Autodesk Fusion 360 part; units mm, degrees
note: some values were not read from the file. Set by a fixed rule: which sketch regions a step uses.
(part 6 of 8)
  spline S324 degree 3 poles (174.1756, -167.163) (173.9248, -167.1552) (173.6715, -167.2604) (173.4975, -167.451) knots 0 0 0 0 1 1 1 1
  spline S325 degree 3 poles (173.4975, -167.451) (173.3234, -167.6416) (173.2329, -167.9153) (173.2621, -168.1781) knots 0 0 0 0 1 1 1 1
  spline S326 degree 3 poles (173.2621, -168.1781) (173.2895, -168.4249) (173.4213, -168.6557) (173.6123, -168.8012) knots 0 0 0 0 1 1 1 1
  spline S327 degree 3 poles (173.6123, -168.8012) (173.8033, -168.9467) (174.0503, -169.0061) (174.283, -168.9676) knots 0 0 0 0 1 1 1 1
  spline S328 degree 3 poles (174.283, -168.9676) (174.4873, -168.9337) (174.6805, -168.8254) (174.8181, -168.6626) knots 0 0 0 0 1 1 1 1
  spline S329 degree 3 poles (174.8181, -168.6626) (174.9557, -168.4998) (175.036, -168.2834) (175.0353, -168.0653) knots 0 0 0 0 1 1 1 1
  spline S330 degree 3 poles (175.0353, -168.0653) (175.0345, -167.8296) (174.9387, -167.5967) (174.7791, -167.4316) knots 0 0 0 0 1 1 1 1
  spline S331 degree 3 poles (174.7791, -167.4316) (174.6196, -167.2666) (174.399, -167.1702) (174.1756, -167.163) knots 0 0 0 0 1 1 1 1
  spline S332 degree 3 poles (194.8527, -168.2399) (194.6019, -168.2321) (194.3486, -168.3373) (194.1746, -168.5279) knots 0 0 0 0 1 1 1 1
  spline S333 degree 3 poles (194.1746, -168.5279) (194.0006, -168.7185) (193.91, -168.9922) (193.9393, -169.255) knots 0 0 0 0 1 1 1 1
  spline S334 degree 3 poles (193.9393, -169.255) (193.9667, -169.5018) (194.0984, -169.7326) (194.2894, -169.8781) knots 0 0 0 0 1 1 1 1
  spline S335 degree 3 poles (194.2894, -169.8781) (194.4804, -170.0236) (194.7274, -170.083) (194.9602, -170.0445) knots 0 0 0 0 1 1 1 1
  spline S336 degree 3 poles (194.9602, -170.0445) (195.1645, -170.0106) (195.3576, -169.9023) (195.4953, -169.7395) knots 0 0 0 0 1 1 1 1
  spline S337 degree 3 poles (195.4953, -169.7395) (195.6328, -169.5767) (195.7131, -169.3603) (195.7124, -169.1422) knots 0 0 0 0 1 1 1 1
  spline S338 degree 3 poles (195.7124, -169.1422) (195.7117, -168.9065) (195.6158, -168.6736) (195.4563, -168.5085) knots 0 0 0 0 1 1 1 1
  spline S339 degree 3 poles (195.4563, -168.5085) (195.2967, -168.3435) (195.0761, -168.2471) (194.8527, -168.2399) knots 0 0 0 0 1 1 1 1
  spline S340 degree 3 poles (211.254, -162.4515) (211.0032, -162.4437) (210.75, -162.5489) (210.5759, -162.7395) knots 0 0 0 0 1 1 1 1
  spline S341 degree 3 poles (210.5759, -162.7395) (210.4019, -162.9302) (210.3114, -163.2038) (210.3406, -163.4666) knots 0 0 0 0 1 1 1 1
  spline S342 degree 3 poles (210.3406, -163.4666) (210.368, -163.7134) (210.4998, -163.9443) (210.6908, -164.0898) knots 0 0 0 0 1 1 1 1
  spline S343 degree 3 poles (210.6908, -164.0898) (210.8818, -164.2353) (211.1287, -164.2946) (211.3615, -164.2561) knots 0 0 0 0 1 1 1 1
  spline S344 degree 3 poles (211.3615, -164.2561) (211.5658, -164.2223) (211.759, -164.1139) (211.8966, -163.9511) knots 0 0 0 0 1 1 1 1
  spline S345 degree 3 poles (211.8966, -163.9511) (212.0342, -163.7884) (212.1144, -163.5719) (212.1137, -163.3538) knots 0 0 0 0 1 1 1 1
  spline S346 degree 3 poles (212.1137, -163.3538) (212.113, -163.1181) (212.0171, -162.8853) (211.8576, -162.7202) knots 0 0 0 0 1 1 1 1
  spline S347 degree 3 poles (211.8576, -162.7202) (211.698, -162.5551) (211.4774, -162.4587) (211.254, -162.4515) knots 0 0 0 0 1 1 1 1
  spline S348 degree 3 poles (210.4882, -175.711) (210.2374, -175.7031) (209.9841, -175.8083) (209.8101, -175.9989) knots 0 0 0 0 1 1 1 1
  spline S349 degree 3 poles (209.8101, -175.9989) (209.6361, -176.1896) (209.5455, -176.4632) (209.5748, -176.726) knots 0 0 0 0 1 1 1 1
  spline S350 degree 3 poles (209.5748, -176.726) (209.6022, -176.9728) (209.7339, -177.2037) (209.9249, -177.3492) knots 0 0 0 0 1 1 1 1
  spline S351 degree 3 poles (209.9249, -177.3492) (210.1159, -177.4947) (210.3629, -177.554) (210.5957, -177.5155) knots 0 0 0 0 1 1 1 1
  spline S352 degree 3 poles (210.5957, -177.5155) (210.8, -177.4817) (210.9931, -177.3733) (211.1307, -177.2106) knots 0 0 0 0 1 1 1 1
  spline S353 degree 3 poles (211.1307, -177.2106) (211.2683, -177.0478) (211.3486, -176.8313) (211.3479, -176.6132) knots 0 0 0 0 1 1 1 1
  spline S354 degree 3 poles (211.3479, -176.6132) (211.3471, -176.3775) (211.2513, -176.1447) (211.0917, -175.9796) knots 0 0 0 0 1 1 1 1
  spline S355 degree 3 poles (211.0917, -175.9796) (210.9322, -175.8145) (210.7116, -175.7181) (210.4882, -175.711) knots 0 0 0 0 1 1 1 1
  line L95 (197.7587, -166.6574) -> (197.7587, -165.3786)
  line L96 (197.7587, -165.3786) -> (207.3315, -165.6478)
  spline S356 degree 3 poles (207.3315, -165.6478) (208.1185, -165.9345) (208.8155, -166.489) (209.2929, -167.2084) knots 0 0 0 0 1 1 1 1
  spline S357 degree 3 poles (209.2929, -167.2084) (209.7704, -167.9277) (210.0258, -168.8082) (210.0119, -169.6862) knots 0 0 0 0 1 1 1 1
  spline S358 degree 3 poles (210.0119, -169.6862) (209.9996, -170.4556) (209.7819, -171.2202) (209.3902, -171.8694) knots 0 0 0 0 1 1 1 1
  spline S359 degree 3 poles (209.3902, -171.8694) (208.9984, -172.5186) (208.4339, -173.0505) (207.7782, -173.3881) knots 0 0 0 0 1 1 1 1
  line L97 (207.7782, -173.3881) -> (197.6949, -173.2534)
  line L98 (197.6949, -173.2534) -> (197.6311, -171.84)
  line L99 (197.6311, -171.84) -> (199.2904, -171.9073)
  line L100 (199.2904, -171.9073) -> (199.2904, -166.792)
  line L101 (199.2904, -166.792) -> (197.7587, -166.6574)
  line L102 (171.183, -170.5055) -> (171.183, -171.7666)
  line L103 (171.183, -171.7666) -> (161.8583, -171.5011)
  spline S360 degree 3 poles (161.8583, -171.5011) (161.0896, -171.2101) (160.4112, -170.6602) (159.9467, -169.9518) knots 0 0 0 0 1 1 1 1
  spline S361 degree 3 poles (159.9467, -169.9518) (159.4823, -169.2433) (159.2341, -168.3798) (159.2473, -167.5186) knots 0 0 0 0 1 1 1 1
  spline S362 degree 3 poles (159.2473, -167.5186) (159.259, -166.7632) (159.4705, -166.0123) (159.8517, -165.3727) knots 0 0 0 0 1 1 1 1
  spline S363 degree 3 poles (159.8517, -165.3727) (160.2329, -164.733) (160.7828, -164.2065) (161.4231, -163.8679) knots 0 0 0 0 1 1 1 1
  line L104 (161.4231, -163.8679) -> (171.2452, -164.0006)
  line L105 (171.2452, -164.0006) -> (171.3073, -165.3945)
  line L106 (171.3073, -165.3945) -> (169.691, -165.3281)
  line L107 (169.691, -165.3281) -> (169.691, -170.3727)
  line L108 (169.691, -170.3727) -> (171.183, -170.5055)
  spline S364 degree 3 poles (232.2093, -186.4811) (232.0787, -186.485) (231.9476, -186.4582) (231.8325, -186.4091) knots 0 0 0 0 1 1 1 1
  spline S365 degree 3 poles (231.8325, -186.4091) (231.7173, -186.3599) (231.6182, -186.2884) (231.5413, -186.2044) knots 0 0 0 0 1 1 1 1
  spline S366 degree 3 poles (231.5413, -186.2044) (231.3875, -186.0364) (231.3261, -185.8227) (231.3347, -185.6151) knots 0 0 0 0 1 1 1 1
  spline S367 degree 3 poles (231.3347, -185.6151) (231.3433, -185.4114) (231.4191, -185.2054) (231.5806, -185.0472) knots 0 0 0 0 1 1 1 1
  spline S368 degree 3 poles (231.5806, -185.0472) (231.6615, -184.9681) (231.7629, -184.9019) (231.8784, -184.8577) knots 0 0 0 0 1 1 1 1
  spline S369 degree 3 poles (231.8784, -184.8577) (231.994, -184.8134) (232.1236, -184.7917) (232.2515, -184.7986) knots 0 0 0 0 1 1 1 1
  spline S370 degree 3 poles (232.2515, -184.7986) (232.3753, -184.8054) (232.4962, -184.839) (232.6008, -184.892) knots 0 0 0 0 1 1 1 1
  spline S371 degree 3 poles (232.6008, -184.892) (232.7055, -184.945) (232.7941, -185.0172) (232.8622, -185.0997) knots 0 0 0 0 1 1 1 1
  spline S372 degree 3 poles (232.8622, -185.0997) (232.9984, -185.2647) (233.0502, -185.4674) (233.0418, -185.6646) knots 0 0 0 0 1 1 1 1
  spline S373 degree 3 poles (233.0418, -185.6646) (233.0332, -185.8575) (232.9676, -186.0524) (232.8236, -186.2078) knots 0 0 0 0 1 1 1 1
  spline S374 degree 3 poles (232.8236, -186.2078) (232.7516, -186.2855) (232.6607, -186.3525) (232.5554, -186.4006) knots 0 0 0 0 1 1 1 1
  spline S375 degree 3 poles (232.5554, -186.4006) (232.4502, -186.4488) (232.3307, -186.4778) (232.2093, -186.4811) knots 0 0 0 0 1 1 1 1
  line L109 (227.6589, -168.8588) -> (226.7503, -182.3862)
  spline S376 degree 3 poles (226.7503, -182.3862) (226.7201, -182.7001) (226.8342, -183.0214) (227.0661, -183.2766) knots 0 0 0 0 1 1 1 1
  spline S377 degree 3 poles (227.0661, -183.2766) (227.2917, -183.5246) (227.6269, -183.7085) (227.9987, -183.788) knots 0 0 0 0 1 1 1 1
  line L110 (227.9987, -183.788) -> (237.2483, -184.5544)
  spline S378 degree 3 poles (237.2483, -184.5544) (237.4241, -184.5476) (237.5976, -184.5046) (237.7473, -184.431) knots 0 0 0 0 1 1 1 1
  spline S379 degree 3 poles (237.7473, -184.431) (237.897, -184.3574) (238.0227, -184.2531) (238.1089, -184.1311) knots 0 0 0 0 1 1 1 1
  spline S380 degree 3 poles (238.1089, -184.1311) (238.261, -183.9159) (238.2873, -183.6607) (238.3138, -183.4147) knots 0 0 0 0 1 1 1 1
  spline S381 degree 3 poles (238.3138, -183.4147) (238.686, -179.9549) (239.0139, -176.4921) (239.2973, -173.0269) knots 0 0 0 0 1 1 1 1
  spline S382 degree 3 poles (239.2973, -173.0269) (239.6327, -168.9267) (239.9059, -164.8233) (240.1169, -160.7179) knots 0 0 0 0 1 1 1 1
  spline S383 degree 3 poles (240.1169, -160.7179) (240.1255, -160.5102) (240.0274, -160.3011) (239.8506, -160.148) knots 0 0 0 0 1 1 1 1
  spline S384 degree 3 poles (239.8506, -160.148) (239.668, -159.99) (239.4033, -159.8938) (239.1334, -159.8875) knots 0 0 0 0 1 1 1 1
  line L111 (239.1334, -159.8875) -> (229.1957, -159.4316)
  spline S385 degree 3 poles (229.1957, -159.4316) (228.874, -159.4703) (228.579, -159.6307) (228.4171, -159.855) knots 0 0 0 0 1 1 1 1
  spline S386 degree 3 poles (228.4171, -159.855) (228.3177, -159.9926) (228.2674, -160.1523) (228.2736, -160.3108) knots 0 0 0 0 1 1 1 1
  line L112 (228.2736, -160.3108) -> (228.1302, -163.0217)
  line L113 (228.1302, -163.0217) -> (227.157, -163.0339)
  spline S387 degree 3 poles (227.157, -163.0339) (227.062, -163.0349) (226.9664, -163.0378) (226.8736, -163.0542) knots 0 0 0 0 1 1 1 1
  spline S388 degree 3 poles (226.8736, -163.0542) (226.7809, -163.0707) (226.6916, -163.1005) (226.6139, -163.144) knots 0 0 0 0 1 1 1 1
  spline S389 degree 3 poles (226.6139, -163.144) (226.4429, -163.2396) (226.3333, -163.4012) (226.3271, -163.5673) knots 0 0 0 0 1 1 1 1
  line L114 (226.3271, -163.5673) -> (225.9787, -168.1425)
  spline S390 degree 3 poles (225.9787, -168.1425) (226.01, -168.2637) (226.0773, -168.3789) (226.1735, -168.4761) knots 0 0 0 0 1 1 1 1
  spline S391 degree 3 poles (226.1735, -168.4761) (226.2642, -168.5679) (226.3805, -168.6435) (226.5115, -168.6961) knots 0 0 0 0 1 1 1 1
  line L115 (226.5115, -168.6961) -> (227.6589, -168.8588)
  spline S392 degree 3 poles (224.9062, -160.356) (224.2581, -164.7818) (223.885, -169.233) (223.7889, -173.688) knots 0 0 0 0 1 1 1 1
  spline S393 degree 3 poles (223.7889, -173.688) (223.693, -178.1315) (223.8093, -182.576) (223.8307, -187.02) knots 0 0 0 0 1 1 1 1
  line L116 (223.8307, -187.02) -> (223.9723, -216.263)
  spline S394 degree 3 poles (223.9723, -216.263) (224.0231, -216.1601) (224.1235, -216.0732) (224.2482, -216.0243) knots 0 0 0 0 1 1 1 1
  spline S395 degree 3 poles (224.2482, -216.0243) (224.373, -215.9754) (224.5208, -215.965) (224.6544, -215.9957) knots 0 0 0 0 1 1 1 1
  spline S396 degree 3 poles (224.6544, -215.9957) (224.8058, -216.0304) (224.9345, -216.1157) (225.0202, -216.2207) knots 0 0 0 0 1 1 1 1
  spline S397 degree 3 poles (225.0202, -216.2207) (225.106, -216.3257) (225.151, -216.4494) (225.1677, -216.5739) knots 0 0 0 0 1 1 1 1
  spline S398 degree 3 poles (225.1677, -216.5739) (225.2012, -216.8228) (225.1259, -217.0718) (225.0962, -217.321) knots 0 0 0 0 1 1 1 1
  spline S399 degree 3 poles (225.0962, -217.321) (225.0221, -217.9422) (225.2425, -218.5829) (225.7041, -219.0877) knots 0 0 0 0 1 1 1 1
  spline S400 degree 3 poles (225.7041, -219.0877) (225.7417, -218.8946) (225.9077, -218.7202) (226.1313, -218.639) knots 0 0 0 0 1 1 1 1
  spline S401 degree 3 poles (226.1313, -218.639) (226.355, -218.5578) (226.6295, -218.5723) (226.8378, -218.6762) knots 0 0 0 0 1 1 1 1
  spline S402 degree 3 poles (226.8378, -218.6762) (226.9476, -218.7309) (227.0382, -218.8081) (227.1089, -218.8945) knots 0 0 0 0 1 1 1 1
  spline S403 degree 3 poles (227.1089, -218.8945) (227.1795, -218.9808) (227.2309, -219.0764) (227.2714, -219.1743) knots 0 0 0 0 1 1 1 1
  spline S404 degree 3 poles (227.2714, -219.1743) (227.3523, -219.3701) (227.3907, -219.5758) (227.4737, -219.771) knots 0 0 0 0 1 1 1 1
  spline S405 degree 3 poles (227.4737, -219.771) (227.6817, -220.261) (228.1819, -220.6668) (228.7939, -220.8424) knots 0 0 0 0 1 1 1 1
  spline S406 degree 3 poles (228.7939, -220.8424) (228.7215, -220.6271) (228.7391, -220.3931) (228.8436, -220.1862) knots 0 0 0 0 1 1 1 1
  spline S407 degree 3 poles (228.8436, -220.1862) (228.9481, -219.9793) (229.1387, -219.8005) (229.3783, -219.6846) knots 0 0 0 0 1 1 1 1
  spline S408 degree 3 poles (229.3783, -219.6846) (229.666, -219.5456) (230.0304, -219.5002) (230.3485, -219.588) knots 0 0 0 0 1 1 1 1
  spline S409 degree 3 poles (230.3485, -219.588) (230.5755, -219.6507) (230.7726, -219.7794) (230.894, -219.9442) knots 0 0 0 0 1 1 1 1
  spline S410 degree 3 poles (230.894, -219.9442) (231.0153, -220.109) (231.06, -220.3085) (231.0176, -220.4965) knots 0 0 0 0 1 1 1 1
  spline S411 degree 3 poles (231.0176, -220.4965) (231.399, -220.4565) (231.7539, -220.278) (231.9627, -220.0213) knots 0 0 0 0 1 1 1 1
  spline S412 degree 3 poles (231.9627, -220.0213) (232.1768, -219.758) (232.2327, -219.4363) (232.3304, -219.1326) knots 0 0 0 0 1 1 1 1
  spline S413 degree 3 poles (232.3304, -219.1326) (232.3792, -218.9807) (232.4403, -218.83) (232.537, -218.6934) knots 0 0 0 0 1 1 1 1
  spline S414 degree 3 poles (232.537, -218.6934) (232.6337, -218.5568) (232.7683, -218.4341) (232.94, -218.3571) knots 0 0 0 0 1 1 1 1
  spline S415 degree 3 poles (232.94, -218.3571) (233.1694, -218.2541) (233.4593, -218.2411) (233.7018, -218.3229) knots 0 0 0 0 1 1 1 1
  spline S416 degree 3 poles (233.7018, -218.3229) (233.9443, -218.4047) (234.1339, -218.5795) (234.2, -218.7821) knots 0 0 0 0 1 1 1 1
  spline S417 degree 3 poles (234.2, -218.7821) (234.4223, -218.5002) (234.5073, -218.1518) (234.4335, -217.8243) knots 0 0 0 0 1 1 1 1
  spline S418 degree 3 poles (234.4335, -217.8243) (234.3698, -217.5418) (234.196, -217.2842) (234.0477, -217.0225) knots 0 0 0 0 1 1 1 1
  spline S419 degree 3 poles (234.0477, -217.0225) (233.8994, -216.7608) (233.7726, -216.4781) (233.8125, -216.1929) knots 0 0 0 0 1 1 1 1
  spline S420 degree 3 poles (233.8125, -216.1929) (233.8482, -215.9371) (234.024, -215.6956) (234.2852, -215.5436) knots 0 0 0 0 1 1 1 1
  spline S421 degree 3 poles (234.2852, -215.5436) (234.5464, -215.3915) (234.8891, -215.3311) (235.2068, -215.3811) knots 0 0 0 0 1 1 1 1
  spline S422 degree 3 poles (235.2068, -215.3811) (235.2638, -215.0376) (235.1143, -214.676) (234.8118, -214.4264) knots 0 0 0 0 1 1 1 1
  spline S423 degree 3 poles (234.8118, -214.4264) (234.6592, -214.3006) (234.4734, -214.204) (234.2913, -214.1061) knots 0 0 0 0 1 1 1 1
  spline S424 degree 3 poles (234.2913, -214.1061) (234.1093, -214.0081) (233.9271, -213.906) (233.786, -213.7719) knots 0 0 0 0 1 1 1 1
  spline S425 degree 3 poles (233.786, -213.7719) (233.6493, -213.642) (233.555, -213.4842) (233.5148, -213.3179) knots 0 0 0 0 1 1 1 1
  spline S426 degree 3 poles (233.5148, -213.3179) (233.4745, -213.1516) (233.4885, -212.9772) (233.5549, -212.8163) knots 0 0 0 0 1 1 1 1
  spline S427 degree 3 poles (233.5549, -212.8163) (233.6212, -212.6554) (233.74, -212.5083) (233.8964, -212.3932) knots 0 0 0 0 1 1 1 1
  spline S428 degree 3 poles (233.8964, -212.3932) (234.0527, -212.2781) (234.2464, -212.1953) (234.4533, -212.155) knots 0 0 0 0 1 1 1 1
  spline S429 degree 3 poles (234.4533, -212.155) (234.3776, -211.9837) (234.2872, -211.8166) (234.183, -211.6551) knots 0 0 0 0 1 1 1 1
  spline S430 degree 3 poles (234.183, -211.6551) (233.5303, -210.6445) (232.3552, -209.8824) (231.7809, -208.8422) knots 0 0 0 0 1 1 1 1
  spline S431 degree 3 poles (231.7809, -208.8422) (231.2851, -207.944) (231.2866, -206.9141) (231.5335, -205.9531) knots 0 0 0 0 1 1 1 1
  spline S432 degree 3 poles (231.5335, -205.9531) (231.7803, -204.9922) (232.2581, -204.0804) (232.6953, -203.1633) knots 0 0 0 0 1 1 1 1
  spline S433 degree 3 poles (232.6953, -203.1633) (233.4614, -201.5562) (234.1092, -199.9155) (234.8011, -198.2873) knots 0 0 0 0 1 1 1 1
  spline S434 degree 3 poles (234.8011, -198.2873) (236.5126, -194.2596) (238.4993, -190.2944) (239.7468, -186.1605) knots 0 0 0 0 1 1 1 1
  spline S435 degree 3 poles (239.7468, -186.1605) (240.674, -183.0881) (241.1854, -179.9454) (241.5499, -176.7991) knots 0 0 0 0 1 1 1 1
  spline S436 degree 3 poles (241.5499, -176.7991) (242.1887, -171.2862) (242.3813, -165.7406) (242.1261, -160.2081) knots 0 0 0 0 1 1 1 1
  spline S437 degree 3 poles (242.1261, -160.2081) (241.9068, -158.8424) (241.1578, -157.5333) (240.0068, -156.5042) knots 0 0 0 0 1 1 1 1
  spline S438 degree 3 poles (240.0068, -156.5042) (238.8559, -155.4751) (237.3079, -154.7302) (235.6269, -154.3967) knots 0 0 0 0 1 1 1 1
  spline S439 degree 3 poles (235.6269, -154.3967) (233.2297, -153.9211) (230.5827, -154.3101) (228.5581, -155.4355) knots 0 0 0 0 1 1 1 1
  spline S440 degree 3 poles (228.5581, -155.4355) (226.5334, -156.5608) (225.1659, -158.4032) (224.9062, -160.356) knots 0 0 0 0 1 1 1 1
  spline S441 degree 3 poles (229.5936, -215.9494) (229.4411, -215.9533) (229.2882, -215.9209) (229.1557, -215.8607) knots 0 0 0 0 1 1 1 1
  spline S442 degree 3 poles (229.1557, -215.8607) (229.0232, -215.8006) (228.911, -215.7138) (228.8257, -215.6132) knots 0 0 0 0 1 1 1 1
  spline S443 degree 3 poles (228.8257, -215.6132) (228.6551, -215.4122) (228.5949, -215.1618) (228.6051, -214.9195) knots 0 0 0 0 1 1 1 1
  spline S444 degree 3 poles (228.6051, -214.9195) (228.6149, -214.6825) (228.6926, -214.4416) (228.8722, -214.2523) knots 0 0 0 0 1 1 1 1
  spline S445 degree 3 poles (228.8722, -214.2523) (228.962, -214.1576) (229.0766, -214.0771) (229.2091, -214.0227) knots 0 0 0 0 1 1 1 1
  spline S446 degree 3 poles (229.2091, -214.0227) (229.3417, -213.9683) (229.4924, -213.9406) (229.6412, -213.9484) knots 0 0 0 0 1 1 1 1
  spline S447 degree 3 poles (229.6412, -213.9484) (229.7862, -213.9562) (229.9273, -213.9972) (230.0477, -214.0618) knots 0 0 0 0 1 1 1 1
  spline S448 degree 3 poles (230.0477, -214.0618) (230.1682, -214.1263) (230.2683, -214.2137) (230.3437, -214.3124) knots 0 0 0 0 1 1 1 1
  spline S449 degree 3 poles (230.3437, -214.3124) (230.4944, -214.5098) (230.5443, -214.7476) (230.5344, -214.9783) knots 0 0 0 0 1 1 1 1
  spline S450 degree 3 poles (230.5344, -214.9783) (230.5246, -215.2032) (230.4579, -215.4317) (230.2981, -215.6175) knots 0 0 0 0 1 1 1 1
  spline S451 degree 3 poles (230.2981, -215.6175) (230.2182, -215.7104) (230.1156, -215.7916) (229.9949, -215.8505) knots 0 0 0 0 1 1 1 1
  spline S452 degree 3 poles (229.9949, -215.8505) (229.8742, -215.9093) (229.7351, -215.9453) (229.5936, -215.9494) knots 0 0 0 0 1 1 1 1
  spline S453 degree 3 poles (234.6434, -158.7579) (234.5128, -158.7618) (234.3817, -158.735) (234.2666, -158.6858) knots 0 0 0 0 1 1 1 1
  spline S454 degree 3 poles (234.2666, -158.6858) (234.1514, -158.6367) (234.0523, -158.5652) (233.9754, -158.4812) knots 0 0 0 0 1 1 1 1
  spline S455 degree 3 poles (233.9754, -158.4812) (233.8216, -158.3132) (233.7602, -158.0995) (233.7688, -157.8919) knots 0 0 0 0 1 1 1 1
  spline S456 degree 3 poles (233.7688, -157.8919) (233.7773, -157.6882) (233.8531, -157.4822) (234.0147, -157.324) knots 0 0 0 0 1 1 1 1
  spline S457 degree 3 poles (234.0147, -157.324) (234.0956, -157.2448) (234.197, -157.1787) (234.3125, -157.1345) knots 0 0 0 0 1 1 1 1
  spline S458 degree 3 poles (234.3125, -157.1345) (234.4281, -157.0902) (234.5576, -157.0685) (234.6855, -157.0754) knots 0 0 0 0 1 1 1 1
  spline S459 degree 3 poles (234.6855, -157.0754) (234.8094, -157.0822) (234.9303, -157.1158) (235.0349, -157.1688) knots 0 0 0 0 1 1 1 1
  spline S460 degree 3 poles (235.0349, -157.1688) (235.1395, -157.2218) (235.2282, -157.294) (235.2963, -157.3765) knots 0 0 0 0 1 1 1 1
  spline S461 degree 3 poles (235.2963, -157.3765) (235.4325, -157.5415) (235.4843, -157.7442) (235.4759, -157.9414) knots 0 0 0 0 1 1 1 1
  spline S462 degree 3 poles (235.4759, -157.9414) (235.4673, -158.1343) (235.4017, -158.3292) (235.2577, -158.4846) knots 0 0 0 0 1 1 1 1
  spline S463 degree 3 poles (235.2577, -158.4846) (235.1856, -158.5623) (235.0947, -158.6293) (234.9895, -158.6774) knots 0 0 0 0 1 1 1 1
  spline S464 degree 3 poles (234.9895, -158.6774) (234.8843, -158.7256) (234.7647, -158.7546) (234.6434, -158.7579) knots 0 0 0 0 1 1 1 1
  spline S465 degree 3 poles (227.5908, -200.8259) (227.6083, -200.9878) (227.7018, -201.1438) (227.8491, -201.2566) knots 0 0 0 0 1 1 1 1
  spline S466 degree 3 poles (227.8491, -201.2566) (227.9965, -201.3693) (228.1963, -201.4376) (228.4006, -201.4452) knots 0 0 0 0 1 1 1 1
  spline S467 degree 3 poles (228.4006, -201.4452) (228.5795, -201.452) (228.7607, -201.4123) (228.9102, -201.3339) knots 0 0 0 0 1 1 1 1
  spline S468 degree 3 poles (228.9102, -201.3339) (229.0597, -201.2555) (229.1767, -201.1387) (229.2393, -201.0054) knots 0 0 0 0 1 1 1 1
  line L117 (229.2393, -201.0054) -> (234.658, -188.8893)
  spline S469 degree 3 poles (234.658, -188.8893) (234.6959, -188.7185) (234.6569, -188.5375) (234.5495, -188.3865) knots 0 0 0 0 1 1 1 1
  spline S470 degree 3 poles (234.5495, -188.3865) (234.4371, -188.2285) (234.2507, -188.1047) (234.0351, -188.0448) knots 0 0 0 0 1 1 1 1
  line L118 (234.0351, -188.0448) -> (228.5617, -187.6122)
  spline S471 degree 3 poles (228.5617, -187.6122) (228.3722, -187.62) (228.1856, -187.6686) (228.0272, -187.7515) knots 0 0 0 0 1 1 1 1
  spline S472 degree 3 poles (228.0272, -187.7515) (227.7632, -187.8896) (227.5834, -188.1247) (227.5506, -188.3745) knots 0 0 0 0 1 1 1 1
  line L119 (227.5506, -188.3745) -> (227.5908, -200.8259)
  spline S473 degree 2 poles (42.2868, -37.3357) (44.6679, -37.1866) (46.1459, -37.3643) knots 0 0 0 1 1 1
  spline S474 degree 3 poles (46.1459, -37.3643) (46.1336, -38.9702) (46.0073, -41.0582) (46.5437, -41.5833) knots 0 0 0 0 1 1 1 1
  spline S475 degree 3 poles (46.5437, -41.5833) (47.2829, -42.5159) (49.4597, -43.7479) (51.759, -43.5945) knots 0 0 0 0 1 1 1 1
  spline S476 degree 3 poles (51.759, -43.5945) (54.1673, -43.434) (55.5304, -41.4405) (56.3952, -39.8243) knots 0 0 0 0 1 1 1 1
  spline S477 degree 3 poles (56.3952, -39.8243) (56.9698, -38.7504) (57.0179, -37.2523) (56.5268, -36.3258) knots 0 0 0 0 1 1 1 1
  spline S478 degree 3 poles (56.5268, -36.3258) (55.3043, -34.0192) (51.084, -30.618) (49.2463, -30.5751) knots 0 0 0 0 1 1 1 1
  spline S479 degree 3 poles (49.2463, -30.5751) (48.0943, -30.5466) (47.0495, -32.7405) (46.6501, -32.6627) knots 0 0 0 0 1 1 1 1
  spline S480 degree 3 poles (46.6501, -32.6627) (46.1834, -32.5719) (45.859, -32.1982) (45.6061, -31.8739) knots 0 0 0 0 1 1 1 1
  spline S481 degree 3 poles (45.6061, -31.8739) (45.2986, -31.4794) (47.8159, -29.3975) (47.8997, -28.7658) knots 0 0 0 0 1 1 1 1
  spline S482 degree 3 poles (47.8997, -28.7658) (47.9763, -28.1886) (47.7958, -27.8125) (47.6265, -27.6679) knots 0 0 0 0 1 1 1 1
  spline S483 degree 3 poles (47.6265, -27.6679) (47.2928, -27.3826) (46.6003, -27.122) (46.2027, -27.1804) knots 0 0 0 0 1 1 1 1
  spline S484 degree 3 poles (46.2027, -27.1804) (46.082, -27.1966) (45.9466, -27.2692) (45.9156, -27.3633) knots 0 0 0 0 1 1 1 1
  spline S485 degree 2 poles (45.9156, -27.3633) (45.8555, -27.5459) (45.85, -28.5927) knots 0 0 0 1 1 1
  line L120 (45.85, -28.5927) -> (42.3251, -28.6791)
  spline S486 degree 2 poles (42.3251, -28.6791) (42.2543, -27.7829) (42.0973, -27.3008) knots 0 0 0 1 1 1
  spline S487 degree 3 poles (42.0973, -27.3008) (42.0592, -27.1835) (41.8946, -27.0914) (41.7444, -27.0686) knots 0 0 0 0 1 1 1 1
  spline S488 degree 3 poles (41.7444, -27.0686) (41.511, -27.0319) (40.8, -27.289) (40.5387, -27.5865) knots 0 0 0 0 1 1 1 1
  spline S489 degree 3 poles (40.5387, -27.5865) (40.291, -27.8684) (40.33, -28.2666) (40.3538, -28.6072) knots 0 0 0 0 1 1 1 1
  spline S490 degree 3 poles (40.3538, -28.6072) (40.399, -29.2553) (43.1675, -31.4738) (42.9159, -31.8178) knots 0 0 0 0 1 1 1 1
  spline S491 degree 2 poles (42.9159, -31.8178) (42.6515, -32.1792) (41.8279, -32.7271) knots 0 0 0 1 1 1
  spline S492 degree 2 poles (41.8279, -32.7271) (40.3643, -30.4802) (39.2074, -30.5073) knots 0 0 0 1 1 1
  spline S493 degree 3 poles (39.2074, -30.5073) (38.2501, -30.5317) (33.4532, -34.048) (32.5474, -35.699) knots 0 0 0 0 1 1 1 1
  spline S494 degree 3 poles (32.5474, -35.699) (31.3187, -37.9383) (32.5495, -39.9259) (33.0916, -40.7431) knots 0 0 0 0 1 1 1 1
  spline S495 degree 3 poles (33.0916, -40.7431) (33.3686, -41.1607) (35.2173, -43.5307) (37.8353, -43.5361) knots 0 0 0 0 1 1 1 1
  spline S496 degree 3 poles (37.8353, -43.5361) (40.1284, -43.2704) (41.4838, -42.2707) (42.1123, -41.7993) knots 0 0 0 0 1 1 1 1
  spline S497 degree 3 poles (42.1123, -41.7993) (42.6989, -41.3593) (42.2945, -39.3731) (42.2867, -37.3353) knots 0 0 0 0 1 1 1 1
  line L121 (42.2867, -37.3353) -> (42.2868, -37.3357)
  spline S498 degree 3 poles (38.3817, -32.5359) (38.128, -32.5328) (37.8418, -32.7612) (37.8435, -32.9618) knots 0 0 0 0 1 1 1 1
  spline S499 degree 3 poles (37.8435, -32.9618) (37.8452, -33.1611) (38.1328, -33.3804) (38.3844, -33.3784) knots 0 0 0 0 1 1 1 1
  spline S500 degree 3 poles (38.3844, -33.3784) (38.6272, -33.3765) (38.8935, -33.1604) (38.8963, -32.9682) knots 0 0 0 0 1 1 1 1
  spline S501 degree 3 poles (38.8963, -32.9682) (38.8992, -32.7702) (38.6318, -32.5388) (38.3817, -32.5359) knots 0 0 0 0 1 1 1 1
  spline S502 degree 3 poles (40.6148, -34.9125) (40.3611, -34.9095) (40.0749, -35.1378) (40.0766, -35.3385) knots 0 0 0 0 1 1 1 1
  spline S503 degree 3 poles (40.0766, -35.3385) (40.0783, -35.5377) (40.3659, -35.757) (40.6175, -35.755) knots 0 0 0 0 1 1 1 1
  spline S504 degree 3 poles (40.6175, -35.755) (40.8602, -35.7531) (41.1266, -35.5371) (41.1294, -35.3449) knots 0 0 0 0 1 1 1 1
  spline S505 degree 3 poles (41.1294, -35.3449) (41.1323, -35.1469) (40.8649, -34.9154) (40.6148, -34.9125) knots 0 0 0 0 1 1 1 1
  spline S506 degree 3 poles (38.3, -34.8692) (38.0463, -34.8662) (37.7601, -35.0946) (37.7618, -35.2953) knots 0 0 0 0 1 1 1 1
  spline S507 degree 3 poles (37.7618, -35.2953) (37.7635, -35.4945) (38.0512, -35.7138) (38.3027, -35.7118) knots 0 0 0 0 1 1 1 1
  spline S508 degree 3 poles (38.3027, -35.7118) (38.5455, -35.7099) (38.8118, -35.4938) (38.8147, -35.3017) knots 0 0 0 0 1 1 1 1
  spline S509 degree 3 poles (38.8147, -35.3017) (38.8176, -35.1036) (38.5501, -34.8722) (38.3, -34.8692) knots 0 0 0 0 1 1 1 1
  spline S510 degree 3 poles (35.8218, -34.6316) (35.5681, -34.6286) (35.2819, -34.8569) (35.2837, -35.0576) knots 0 0 0 0 1 1 1 1
  spline S511 degree 3 poles (35.2837, -35.0576) (35.2854, -35.2569) (35.573, -35.4762) (35.8245, -35.4742) knots 0 0 0 0 1 1 1 1
  spline S512 degree 3 poles (35.8245, -35.4742) (36.0673, -35.4723) (36.3336, -35.2562) (36.3365, -35.064) knots 0 0 0 0 1 1 1 1
  spline S513 degree 3 poles (36.3365, -35.064) (36.3394, -34.866) (36.072, -34.6346) (35.8218, -34.6316) knots 0 0 0 0 1 1 1 1
  spline S514 degree 3 poles (36.2848, -37.6565) (36.0311, -37.6534) (35.7449, -37.8818) (35.7466, -38.0825) knots 0 0 0 0 1 1 1 1
  spline S515 degree 3 poles (35.7466, -38.0825) (35.7483, -38.2817) (36.0359, -38.501) (36.2875, -38.499) knots 0 0 0 0 1 1 1 1
  spline S516 degree 3 poles (36.2875, -38.499) (36.5303, -38.4972) (36.7966, -38.2811) (36.7995, -38.089) knots 0 0 0 0 1 1 1 1
  spline S517 degree 3 poles (36.7995, -38.089) (36.8023, -37.8909) (36.5349, -37.6595) (36.2848, -37.6565) knots 0 0 0 0 1 1 1 1
  spline S518 degree 3 poles (38.5723, -37.6996) (38.3186, -37.6966) (38.0324, -37.9249) (38.0342, -38.1256) knots 0 0 0 0 1 1 1 1
  spline S519 degree 3 poles (38.0342, -38.1256) (38.0358, -38.3249) (38.3235, -38.5442) (38.575, -38.5422) knots 0 0 0 0 1 1 1 1
  spline S520 degree 3 poles (38.575, -38.5422) (38.8178, -38.5403) (39.0841, -38.3242) (39.087, -38.132) knots 0 0 0 0 1 1 1 1
  spline S521 degree 3 poles (39.087, -38.132) (39.0899, -37.934) (38.8225, -37.7026) (38.5723, -37.6996) knots 0 0 0 0 1 1 1 1
  spline S522 degree 3 poles (40.996, -37.5052) (40.7423, -37.5022) (40.4561, -37.7305) (40.4579, -37.9312) knots 0 0 0 0 1 1 1 1
  spline S523 degree 3 poles (40.4579, -37.9312) (40.4596, -38.1305) (40.7472, -38.3498) (40.9987, -38.3478) knots 0 0 0 0 1 1 1 1
  spline S524 degree 3 poles (40.9987, -38.3478) (41.2415, -38.3459) (41.5078, -38.1298) (41.5107, -37.9376) knots 0 0 0 0 1 1 1 1
  spline S525 degree 3 poles (41.5107, -37.9376) (41.5136, -37.7396) (41.2462, -37.5082) (40.996, -37.5052) knots 0 0 0 0 1 1 1 1
  spline S526 degree 3 poles (34.0245, -37.2027) (33.7708, -37.1996) (33.4846, -37.428) (33.4863, -37.6287) knots 0 0 0 0 1 1 1 1
  spline S527 degree 3 poles (33.4863, -37.6287) (33.488, -37.8279) (33.7756, -38.0472) (34.0272, -38.0452) knots 0 0 0 0 1 1 1 1
  spline S528 degree 3 poles (34.0272, -38.0452) (34.27, -38.0433) (34.5363, -37.8273) (34.5391, -37.6351) knots 0 0 0 0 1 1 1 1
  spline S529 degree 3 poles (34.5391, -37.6351) (34.542, -37.4371) (34.2746, -37.2057) (34.0245, -37.2027) knots 0 0 0 0 1 1 1 1
  spline S530 degree 3 poles (35.7946, -40.3572) (35.5409, -40.3542) (35.2547, -40.5825) (35.2564, -40.7832) knots 0 0 0 0 1 1 1 1
  spline S531 degree 3 poles (35.2564, -40.7832) (35.2581, -40.9824) (35.5457, -41.2017) (35.7973, -41.1997) knots 0 0 0 0 1 1 1 1
  spline S532 degree 3 poles (35.7973, -41.1997) (36.0401, -41.1978) (36.3064, -40.9817) (36.3092, -40.7896) knots 0 0 0 0 1 1 1 1
  spline S533 degree 3 poles (36.3092, -40.7896) (36.3122, -40.5915) (36.0447, -40.3601) (35.7946, -40.3572) knots 0 0 0 0 1 1 1 1
  spline S534 degree 3 poles (37.9187, -40.3356) (37.665, -40.3325) (37.3788, -40.5609) (37.3806, -40.7616) knots 0 0 0 0 1 1 1 1
  spline S535 degree 3 poles (37.3806, -40.7616) (37.3823, -40.9609) (37.6699, -41.1801) (37.9214, -41.1782) knots 0 0 0 0 1 1 1 1
  spline S536 degree 3 poles (37.9214, -41.1782) (38.1642, -41.1762) (38.4305, -40.9602) (38.4334, -40.768) knots 0 0 0 0 1 1 1 1
  spline S537 degree 3 poles (38.4334, -40.768) (38.4363, -40.57) (38.1689, -40.3386) (37.9187, -40.3356) knots 0 0 0 0 1 1 1 1
  spline S538 degree 3 poles (40.3424, -39.9467) (40.0888, -39.9436) (39.8025, -40.172) (39.8043, -40.3726) knots 0 0 0 0 1 1 1 1
  spline S539 degree 3 poles (39.8043, -40.3726) (39.806, -40.5719) (40.0936, -40.7912) (40.3452, -40.7892) knots 0 0 0 0 1 1 1 1
  spline S540 degree 3 poles (40.3452, -40.7892) (40.5879, -40.7873) (40.8542, -40.5712) (40.8571, -40.379) knots 0 0 0 0 1 1 1 1
  spline S541 degree 3 poles (40.8571, -40.379) (40.86, -40.181) (40.5926, -39.9496) (40.3424, -39.9467) knots 0 0 0 0 1 1 1 1
  spline S542 degree 3 poles (49.8194, -32.5575) (49.5657, -32.5544) (49.2795, -32.7828) (49.2813, -32.9835) knots 0 0 0 0 1 1 1 1
  spline S543 degree 3 poles (49.2813, -32.9835) (49.2829, -33.1827) (49.5706, -33.402) (49.8221, -33.4) knots 0 0 0 0 1 1 1 1
  spline S544 degree 3 poles (49.8221, -33.4) (50.0649, -33.3981) (50.3312, -33.1821) (50.3341, -32.9899) knots 0 0 0 0 1 1 1 1
  spline S545 degree 3 poles (50.3341, -32.9899) (50.337, -32.7919) (50.0696, -32.5604) (49.8194, -32.5575) knots 0 0 0 0 1 1 1 1
  spline S546 degree 3 poles (47.4774, -34.8477) (47.2237, -34.8446) (46.9375, -35.073) (46.9392, -35.2736) knots 0 0 0 0 1 1 1 1
  spline S547 degree 3 poles (46.9392, -35.2736) (46.9409, -35.4729) (47.2286, -35.6922) (47.4801, -35.6902) knots 0 0 0 0 1 1 1 1
  spline S548 degree 3 poles (47.4801, -35.6902) (47.7229, -35.6883) (47.9892, -35.4722) (47.9921, -35.28) knots 0 0 0 0 1 1 1 1
  spline S549 degree 3 poles (47.9921, -35.28) (47.995, -35.082) (47.7275, -34.8506) (47.4774, -34.8477) knots 0 0 0 0 1 1 1 1
  spline S550 degree 3 poles (49.9011, -34.8692) (49.6474, -34.8662) (49.3612, -35.0946) (49.3629, -35.2953) knots 0 0 0 0 1 1 1 1
  spline S551 degree 3 poles (49.3629, -35.2953) (49.3646, -35.4945) (49.6522, -35.7138) (49.9038, -35.7118) knots 0 0 0 0 1 1 1 1
  spline S552 degree 3 poles (49.9038, -35.7118) (50.1466, -35.7099) (50.4129, -35.4938) (50.4158, -35.3017) knots 0 0 0 0 1 1 1 1
  spline S553 degree 3 poles (50.4158, -35.3017) (50.4187, -35.1036) (50.1512, -34.8722) (49.9011, -34.8692) knots 0 0 0 0 1 1 1 1
  spline S554 degree 3 poles (52.0252, -34.6748) (51.7716, -34.6718) (51.4853, -34.9001) (51.4871, -35.1008) knots 0 0 0 0 1 1 1 1
  spline S555 degree 3 poles (51.4871, -35.1008) (51.4888, -35.3) (51.7764, -35.5193) (52.028, -35.5173) knots 0 0 0 0 1 1 1 1
  spline S556 degree 3 poles (52.028, -35.5173) (52.2707, -35.5154) (52.537, -35.2994) (52.5399, -35.1072) knots 0 0 0 0 1 1 1 1
  spline S557 degree 3 poles (52.5399, -35.1072) (52.5428, -34.9092) (52.2754, -34.6778) (52.0252, -34.6748) knots 0 0 0 0 1 1 1 1
  spline S558 degree 3 poles (47.2868, -37.462) (47.0331, -37.4589) (46.7469, -37.6873) (46.7486, -37.8879) knots 0 0 0 0 1 1 1 1
  spline S559 degree 3 poles (46.7486, -37.8879) (46.7503, -38.0872) (47.0379, -38.3065) (47.2895, -38.3045) knots 0 0 0 0 1 1 1 1
  spline S560 degree 3 poles (47.2895, -38.3045) (47.5322, -38.3026) (47.7986, -38.0865) (47.8014, -37.8943) knots 0 0 0 0 1 1 1 1
  spline S561 degree 3 poles (47.8014, -37.8943) (47.8043, -37.6963) (47.5369, -37.4649) (47.2868, -37.462) knots 0 0 0 0 1 1 1 1
  spline S562 degree 3 poles (47.8586, -39.7738) (47.605, -39.7708) (47.3187, -39.9992) (47.3205, -40.1998) knots 0 0 0 0 1 1 1 1
  spline S563 degree 3 poles (47.3205, -40.1998) (47.3222, -40.3991) (47.6098, -40.6183) (47.8614, -40.6164) knots 0 0 0 0 1 1 1 1
  spline S564 degree 3 poles (47.8614, -40.6164) (48.1041, -40.6144) (48.3704, -40.3984) (48.3733, -40.2062) knots 0 0 0 0 1 1 1 1
  spline S565 degree 3 poles (48.3733, -40.2062) (48.3762, -40.0082) (48.1088, -39.7768) (47.8586, -39.7738) knots 0 0 0 0 1 1 1 1
  spline S566 degree 3 poles (49.7105, -37.678) (49.4568, -37.675) (49.1706, -37.9034) (49.1723, -38.1041) knots 0 0 0 0 1 1 1 1
  spline S567 degree 3 poles (49.1723, -38.1041) (49.174, -38.3033) (49.4616, -38.5226) (49.7132, -38.5206) knots 0 0 0 0 1 1 1 1
  spline S568 degree 3 poles (49.7132, -38.5206) (49.956, -38.5187) (50.2223, -38.3026) (50.2252, -38.1105) knots 0 0 0 0 1 1 1 1
  spline S569 degree 3 poles (50.2252, -38.1105) (50.228, -37.9124) (49.9606, -37.681) (49.7105, -37.678) knots 0 0 0 0 1 1 1 1
  spline S570 degree 3 poles (49.7105, -37.678) (49.4568, -37.675) (49.1706, -37.9034) (49.1723, -38.1041) knots 0 0 0 0 1 1 1 1
  spline S571 degree 3 poles (49.1723, -38.1041) (49.174, -38.3033) (49.4616, -38.5226) (49.7132, -38.5206) knots 0 0 0 0 1 1 1 1
  spline S572 degree 3 poles (49.7132, -38.5206) (49.956, -38.5187) (50.2223, -38.3026) (50.2252, -38.1105) knots 0 0 0 0 1 1 1 1
  spline S573 degree 3 poles (50.2252, -38.1105) (50.228, -37.9124) (49.9606, -37.681) (49.7105, -37.678) knots 0 0 0 0 1 1 1 1
  spline S574 degree 3 poles (50.0373, -40.4652) (49.7836, -40.4622) (49.4974, -40.6905) (49.4991, -40.8912) knots 0 0 0 0 1 1 1 1
  spline S575 degree 3 poles (49.4991, -40.8912) (49.5008, -41.0905) (49.7884, -41.3098) (50.04, -41.3078) knots 0 0 0 0 1 1 1 1
  spline S576 degree 3 poles (50.04, -41.3078) (50.2828, -41.3059) (50.5491, -41.0898) (50.5519, -40.8976) knots 0 0 0 0 1 1 1 1
  spline S577 degree 3 poles (50.5519, -40.8976) (50.5548, -40.6996) (50.2874, -40.4681) (50.0373, -40.4652) knots 0 0 0 0 1 1 1 1
  spline S578 degree 3 poles (52.5699, -40.4436) (52.3162, -40.4406) (52.03, -40.669) (52.0317, -40.8696) knots 0 0 0 0 1 1 1 1
  spline S579 degree 3 poles (52.0317, -40.8696) (52.0334, -41.0689) (52.3211, -41.2881) (52.5726, -41.2861) knots 0 0 0 0 1 1 1 1
  spline S580 degree 3 poles (52.5726, -41.2861) (52.8154, -41.2842) (53.0817, -41.0682) (53.0846, -40.876) knots 0 0 0 0 1 1 1 1
  spline S581 degree 3 poles (53.0846, -40.876) (53.0874, -40.678) (52.82, -40.4466) (52.5699, -40.4436) knots 0 0 0 0 1 1 1 1
  spline S582 degree 3 poles (51.9435, -37.6132) (51.6898, -37.6102) (51.4036, -37.8385) (51.4054, -38.0392) knots 0 0 0 0 1 1 1 1
  spline S583 degree 3 poles (51.4054, -38.0392) (51.4071, -38.2385) (51.6947, -38.4578) (51.9462, -38.4558) knots 0 0 0 0 1 1 1 1
  spline S584 degree 3 poles (51.9462, -38.4558) (52.189, -38.4538) (52.4553, -38.2378) (52.4582, -38.0456) knots 0 0 0 0 1 1 1 1
  spline S585 degree 3 poles (52.4582, -38.0456) (52.4611, -37.8476) (52.1937, -37.6162) (51.9435, -37.6132) knots 0 0 0 0 1 1 1 1
  spline S586 degree 3 poles (54.1222, -37.4836) (53.8685, -37.4806) (53.5823, -37.7089) (53.584, -37.9096) knots 0 0 0 0 1 1 1 1
  spline S587 degree 3 poles (53.584, -37.9096) (53.5857, -38.1088) (53.8733, -38.3281) (54.1249, -38.3261) knots 0 0 0 0 1 1 1 1
  spline S588 degree 3 poles (54.1249, -38.3261) (54.3677, -38.3242) (54.634, -38.1082) (54.6368, -37.916) knots 0 0 0 0 1 1 1 1
  spline S589 degree 3 poles (54.6368, -37.916) (54.6397, -37.718) (54.3723, -37.4866) (54.1222, -37.4836) knots 0 0 0 0 1 1 1 1
  spline S590 degree 3 poles (17.6619, -44.0788) (17.5828, -43.878) (17.624, -43.6193) (17.9059, -43.4884) knots 0 0 0 0 1 1 1 1
  line L122 (17.9059, -43.4884) -> (19.6099, -42.6972)
  spline S591 degree 3 poles (19.6099, -42.6972) (19.7738, -42.621) (20.0787, -42.6505) (20.1953, -42.8082) knots 0 0 0 0 1 1 1 1
  spline S592 degree 2 poles (20.1953, -42.8082) (23.6928, -47.2967) (24.919, -48.5889) knots 0 0 0 1 1 1
  spline S593 degree 3 poles (24.919, -48.5889) (25.968, -49.6942) (27.2329, -50.4227) (28.7236, -50.4977) knots 0 0 0 0 1 1 1 1
  spline S594 degree 2 poles (28.7236, -50.4977) (31.8275, -50.6538) (41.7276, -50.0288) knots 0 0 0 1 1 1
  spline S595 degree 3 poles (41.7276, -50.0288) (42.5967, -49.9993) (42.3943, -47.6516) (41.7262, -47.6534) knots 0 0 0 0 1 1 1 1
  line L123 (41.7262, -47.6534) -> (35.4954, -47.6703)
  spline S596 degree 3 poles (35.4954, -47.6703) (35.2464, -47.6709) (35.1663, -47.5777) (35.1635, -47.245) knots 0 0 0 0 1 1 1 1
  line L124 (35.1635, -47.245) -> (35.1475, -45.3596)
  spline S597 degree 3 poles (35.1475, -45.3596) (35.1452, -45.0903) (35.0803, -44.9838) (34.743, -44.9813) knots 0 0 0 0 1 1 1 1
  line L125 (34.743, -44.9813) -> (31.0423, -44.9518)
  spline S598 degree 3 poles (31.0423, -44.9518) (30.6787, -44.949) (30.5999, -44.8373) (30.6055, -44.321) knots 0 0 0 0 1 1 1 1
  line L126 (30.6055, -44.321) -> (30.6835, -37.1182)
  spline S599 degree 3 poles (30.6835, -37.1182) (30.6935, -36.1876) (28.6106, -35.6774) (28.5253, -33.4993) knots 0 0 0 0 1 1 1 1
  spline S600 degree 3 poles (28.5253, -33.4993) (28.3933, -30.129) (31.3849, -29.8142) (31.383, -28.7843) knots 0 0 0 0 1 1 1 1
  line L127 (31.383, -28.7843) -> (31.3782, -26.1762)
  spline S601 degree 3 poles (31.3782, -26.1762) (31.3778, -25.9666) (31.5395, -25.9305) (31.6624, -25.9283) knots 0 0 0 0 1 1 1 1
  line L128 (31.6624, -25.9283) -> (34.4801, -25.8774)
  spline S602 degree 3 poles (34.4801, -25.8774) (34.604, -25.8752) (34.7281, -25.9692) (34.7298, -26.1001) knots 0 0 0 0 1 1 1 1
  line L129 (34.7298, -26.1001) -> (34.7462, -27.3313)
  spline S603 degree 3 poles (34.7462, -27.3313) (34.7487, -27.806) (34.9557, -27.8929) (35.273, -27.9133) knots 0 0 0 0 1 1 1 1
  spline S604 degree 2 poles (35.273, -27.9133) (37.2602, -27.8923) (37.2747, -27.9049) knots 0 0 0 1 1 1
  spline S605 degree 3 poles (37.2747, -27.9049) (37.4639, -27.9007) (37.4877, -27.7968) (37.491, -27.6933) knots 0 0 0 0 1 1 1 1
  line L130 (37.491, -27.6933) -> (37.501, -27.3768)
  spline S606 degree 3 poles (37.501, -27.3768) (37.4962, -27.1601) (37.6116, -27.1618) (37.7928, -27.1614) knots 0 0 0 0 1 1 1 1
  line L131 (37.7928, -27.1614) -> (41.0021, -27.153)
  spline S607 degree 3 poles (41.0021, -27.153) (41.2473, -27.1523) (41.4821, -27.1151) (41.5142, -26.7355) knots 0 0 0 0 1 1 1 1
  line L132 (41.5142, -26.7355) -> (41.4903, -22.0584)
  spline S608 degree 3 poles (41.4903, -22.0584) (41.4881, -21.6273) (41.5416, -21.5678) (41.9417, -21.5743) knots 0 0 0 0 1 1 1 1
  spline S609 degree 2 poles (41.9417, -21.5743) (43.9635, -21.4519) (44.5677, -21.7452) knots 0 0 0 1 1 1
  spline S610 degree 3 poles (44.5677, -21.7452) (44.865, -21.8896) (47.3706, -25.0219) (48.1014, -26.7255) knots 0 0 0 0 1 1 1 1
  spline S611 degree 3 poles (48.1014, -26.7255) (48.781, -28.3096) (49.0045, -28.5976) (50.631, -28.5556) knots 0 0 0 0 1 1 1 1
  spline S612 degree 2 poles (50.631, -28.5556) (51.8882, -28.5219) (55.6772, -28.4399) knots 0 0 0 1 1 1
  spline S613 degree 3 poles (55.6772, -28.4399) (56.137, -28.4356) (56.3218, -28.5501) (56.3415, -28.9948) knots 0 0 0 0 1 1 1 1
  line L133 (56.3415, -28.9948) -> (56.4801, -32.1163)
  spline S614 degree 3 poles (56.4801, -32.1163) (56.4767, -32.772) (56.8347, -32.9776) (57.3102, -32.9322) knots 0 0 0 0 1 1 1 1
  line L134 (57.3102, -32.9322) -> (58.4043, -32.9027)
  spline S615 degree 3 poles (58.4043, -32.9027) (58.9625, -32.8732) (59.33, -33.0652) (59.3481, -33.7413) knots 0 0 0 0 1 1 1 1
  line L135 (59.3481, -33.7413) -> (59.7119, -47.3789)
  spline S616 degree 3 poles (59.7119, -47.3789) (59.7199, -47.6453) (59.7778, -47.8415) (59.4228, -47.8594) knots 0 0 0 0 1 1 1 1
  line L136 (59.4228, -47.8594) -> (57.5417, -47.9541)
  spline S617 degree 3 poles (57.5417, -47.9541) (57.2829, -47.9668) (57.1248, -48.1595) (57.1287, -48.4321) knots 0 0 0 0 1 1 1 1
  line L137 (57.1287, -48.4321) -> (57.1778, -51.8487)
  spline S618 degree 3 poles (57.1778, -51.8487) (57.1858, -52.4147) (57.0852, -52.5079) (56.7248, -52.527) knots 0 0 0 0 1 1 1 1
  line L138 (56.7248, -52.527) -> (48.3893, -52.971)
  spline S619 degree 3 poles (48.3893, -52.971) (47.6182, -53.0131) (46.3664, -55.2438) (43.9004, -55.3319) knots 0 0 0 0 1 1 1 1
  spline S620 degree 3 poles (43.9004, -55.3319) (41.4519, -55.4194) (41.1997, -53.4012) (40.5699, -53.4379) knots 0 0 0 0 1 1 1 1
  spline S621 degree 2 poles (40.5699, -53.4379) (22.9209, -54.606) (21.7289, -54.3591) knots 0 0 0 1 1 1
  spline S622 degree 2 poles (21.7289, -54.3591) (20.9439, -54.1967) (17.663, -44.0839) knots 0 0 0 1 1 1
  line L139 (17.663, -44.0839) -> (17.6619, -44.0788)
  spline S623 degree 3 poles (15.3571, -42.3987) (15.2531, -44.1928) (19.1965, -57.8769) (24.3635, -60.2198) knots 0 0 0 0 1 1 1 1
  spline S624 degree 3 poles (24.3635, -60.2198) (26.0533, -60.986) (28.7323, -61.2499) (29.6338, -60.8173) knots 0 0 0 0 1 1 1 1
  spline S625 degree 3 poles (29.6338, -60.8173) (37.8076, -56.8954) (43.4008, -58.1457) (51.8545, -58.0114) knots 0 0 0 0 1 1 1 1
  spline S626 degree 3 poles (51.8545, -58.0114) (59.4967, -57.8898) (62.8323, -49.9984) (63.124, -44.2265) knots 0 0 0 0 1 1 1 1
  spline S627 degree 3 poles (63.124, -44.2265) (63.7591, -31.6611) (58.1578, -23.4181) (51.493, -20.3003) knots 0 0 0 0 1 1 1 1
  spline S628 degree 3 poles (51.493, -20.3003) (41.2639, -15.5151) (26.673, -19.8765) (23.1626, -29.7446) knots 0 0 0 0 1 1 1 1
  spline S629 degree 3 poles (23.1626, -29.7446) (22.3637, -31.9906) (22.606, -34.3973) (21.4948, -36.3528) knots 0 0 0 0 1 1 1 1
  spline S630 degree 3 poles (21.4948, -36.3528) (20.0561, -38.8847) (15.4459, -40.8683) (15.3571, -42.3987) knots 0 0 0 0 1 1 1 1
  spline S631 degree 3 poles (50.3366, -26.1217) (50.6607, -26.1219) (51.0421, -26.3994) (51.0411, -26.8278) knots 0 0 0 0 1 1 1 1
  spline S632 degree 3 poles (51.0411, -26.8278) (51.0401, -27.2811) (50.7474, -27.6061) (50.3421, -27.6077) knots 0 0 0 0 1 1 1 1
  spline S633 degree 3 poles (50.3421, -27.6077) (49.9086, -27.6094) (49.5998, -27.2268) (49.5925, -26.8656) knots 0 0 0 0 1 1 1 1
  spline S634 degree 3 poles (49.5925, -26.8656) (49.5834, -26.4183) (49.9039, -26.1215) (50.3366, -26.1217) knots 0 0 0 0 1 1 1 1
  spline S635 degree 3 poles (51.5238, -53.5459) (51.8479, -53.5461) (52.2293, -53.8236) (52.2283, -54.252) knots 0 0 0 0 1 1 1 1
  spline S636 degree 3 poles (52.2283, -54.252) (52.2273, -54.7053) (51.9346, -55.0303) (51.5293, -55.0319) knots 0 0 0 0 1 1 1 1
  spline S637 degree 3 poles (51.5293, -55.0319) (51.0958, -55.0336) (50.787, -54.651) (50.7797, -54.2898) knots 0 0 0 0 1 1 1 1
  spline S638 degree 3 poles (50.7797, -54.2898) (50.7705, -53.8425) (51.0911, -53.5457) (51.5238, -53.5459) knots 0 0 0 0 1 1 1 1
  spline S639 degree 3 poles (72.4077, -14.495) (76.2222, -14.5808) (80.511, -17.3895) (80.5013, -22.9487) knots 0 0 0 0 1 1 1 1
  spline S640 degree 3 poles (80.5013, -22.9487) (80.4933, -27.4799) (76.2714, -30.9917) (72.596, -30.8125) knots 0 0 0 0 1 1 1 1
  spline S641 degree 3 poles (72.596, -30.8125) (67.4474, -30.5616) (64.6157, -26.4626) (64.4083, -22.1623) knots 0 0 0 0 1 1 1 1
  spline S642 degree 3 poles (64.4083, -22.1623) (64.1959, -17.756) (68.7896, -14.4139) (72.4077, -14.495) knots 0 0 0 0 1 1 1 1
  spline S643 degree 3 poles (74.4782, -39.3644) (78.2926, -39.4501) (82.5814, -42.2589) (82.5717, -47.8181) knots 0 0 0 0 1 1 1 1
  spline S644 degree 3 poles (82.5717, -47.8181) (82.5637, -52.3493) (78.3418, -55.861) (74.6664, -55.6819) knots 0 0 0 0 1 1 1 1
  spline S645 degree 3 poles (74.6664, -55.6819) (69.5179, -55.431) (66.6861, -51.332) (66.4788, -47.0317) knots 0 0 0 0 1 1 1 1
  spline S646 degree 3 poles (66.4788, -47.0317) (66.2663, -42.6253) (70.86, -39.2833) (74.4782, -39.3644) knots 0 0 0 0 1 1 1 1
  spline S647 degree 3 poles (73.2547, -58.1885) (82.2738, -57.514) (89.929, -48.2391) (90.0911, -35.5547) knots 0 0 0 0 1 1 1 1
  spline S648 degree 2 poles (90.0911, -35.5547) (87.4582, -35.4186) (84.5732, -35.2996) knots 0 0 0 1 1 1
  line L140 (84.5732, -35.2996) -> (84.4436, -32.0379)
  spline S649 degree 2 poles (84.4436, -32.0379) (87.0133, -31.8148) (89.6301, -31.7957) knots 0 0 0 1 1 1
  spline S650 degree 3 poles (89.6301, -31.7957) (89.3881, -23.0694) (80.8894, -11.9692) (70.8536, -11.9574) knots 0 0 0 0 1 1 1 1
  spline S651 degree 3 poles (70.8536, -11.9574) (65.8926, -11.9533) (60.827, -16.7994) (60.6359, -22.2236) knots 0 0 0 0 1 1 1 1
  spline S652 degree 3 poles (60.6359, -22.2236) (60.4745, -26.8052) (64.4528, -30.3758) (65.4603, -34.4155) knots 0 0 0 0 1 1 1 1
  spline S653 degree 2 poles (65.4603, -34.4155) (66.0969, -34.4488) (67.0164, -34.4149) knots 0 0 0 1 1 1
  line L141 (67.0164, -34.4149) -> (67.0519, -37.0172)
  spline S654 degree 2 poles (67.0519, -37.0172) (65.9687, -37.0863) (65.5157, -37.0863) knots 0 0 0 1 1 1
  spline S655 degree 3 poles (65.5157, -37.0863) (65.3104, -41.7972) (62.9265, -42.7565) (63.0688, -47.555) knots 0 0 0 0 1 1 1 1
  spline S656 degree 3 poles (63.0688, -47.555) (63.2869, -54.9073) (68.8035, -58.284) (73.2547, -58.1885) knots 0 0 0 0 1 1 1 1
  spline S657 degree 3 poles (75.2311, -32.5366) (76.2994, -32.5199) (77.0863, -32.4829) (78.4243, -32.487) knots 0 0 0 0 1 1 1 1
  spline S658 degree 3 poles (78.4243, -32.487) (79.2745, -32.4892) (79.9669, -33.2482) (80.0113, -34.542) knots 0 0 0 0 1 1 1 1
  spline S659 degree 3 poles (80.0113, -34.542) (80.0451, -35.5268) (79.4809, -36.6514) (78.5513, -36.6998) knots 0 0 0 0 1 1 1 1
  spline S660 degree 3 poles (78.5513, -36.6998) (77.2938, -36.7651) (76.3755, -36.7248) (74.8851, -36.7331) knots 0 0 0 0 1 1 1 1
  spline S661 degree 3 poles (74.8851, -36.7331) (73.8536, -36.7373) (73.3473, -35.5264) (73.3497, -34.5799) knots 0 0 0 0 1 1 1 1
  spline S662 degree 3 poles (73.3497, -34.5799) (73.3525, -33.5069) (73.9685, -32.5568) (75.2311, -32.5385) knots 0 0 0 0 1 1 1 1
  line L142 (75.2311, -32.5385) -> (75.2311, -32.5366)
  spline S663 degree 3 poles (23.3609, -72.9778) (22.2129, -71.851) (21.4757, -70.2714) (21.3301, -68.6262) knots 0 0 0 0 1 1 1 1
  spline S664 degree 3 poles (21.3301, -68.6262) (21.2105, -67.2742) (21.5015, -65.8524) (22.2921, -64.7795) knots 0 0 0 0 1 1 1 1
  spline S665 degree 3 poles (22.2921, -64.7795) (22.6874, -64.243) (23.2025, -63.8013) (23.7918, -63.5252) knots 0 0 0 0 1 1 1 1
  spline S666 degree 3 poles (23.7918, -63.5252) (24.381, -63.2491) (25.0442, -63.1419) (25.6819, -63.2439) knots 0 0 0 0 1 1 1 1
  spline S667 degree 3 poles (25.6819, -63.2439) (25.9327, -63.284) (26.179, -63.3559) (26.4137, -63.4575) knots 0 0 0 0 1 1 1 1
  line L143 (26.4137, -63.4575) -> (26.3346, -66.4885)
  spline S668 degree 3 poles (26.3346, -66.4885) (26.3328, -66.559) (26.3313, -66.63) (26.3432, -66.6993) knots 0 0 0 0 1 1 1 1
  spline S669 degree 3 poles (26.3432, -66.6993) (26.3551, -66.7687) (26.3808, -66.8367) (26.4253, -66.8893) knots 0 0 0 0 1 1 1 1
  spline S670 degree 3 poles (26.4253, -66.8893) (26.4752, -66.9483) (26.5458, -66.9845) (26.6187, -67.0028) knots 0 0 0 0 1 1 1 1
  spline S671 degree 3 poles (26.6187, -67.0028) (26.6917, -67.021) (26.7674, -67.0222) (26.8423, -67.0229) knots 0 0 0 0 1 1 1 1
  line L144 (26.8423, -67.0229) -> (30.6138, -67.0611)
  spline S672 degree 3 poles (30.6138, -67.0611) (30.7278, -67.0622) (30.842, -67.0657) (30.9556, -67.0562) knots 0 0 0 0 1 1 1 1
  spline S673 degree 3 poles (30.9556, -67.0562) (31.0692, -67.0467) (31.185, -67.0218) (31.2803, -66.9561) knots 0 0 0 0 1 1 1 1
  spline S674 degree 3 poles (31.2803, -66.9561) (31.3492, -66.9086) (31.405, -66.8402) (31.4393, -66.7614) knots 0 0 0 0 1 1 1 1
  spline S675 degree 3 poles (31.4393, -66.7614) (31.4736, -66.6825) (31.4862, -66.5934) (31.4753, -66.5075) knots 0 0 0 0 1 1 1 1
  line L145 (31.4753, -66.5075) -> (31.5205, -64.1219)
  spline S676 degree 3 poles (31.5205, -64.1219) (31.5016, -64.0446) (31.5043, -63.9616) (31.5283, -63.8859) knots 0 0 0 0 1 1 1 1
  spline S677 degree 3 poles (31.5283, -63.8859) (31.5523, -63.8102) (31.5974, -63.7421) (31.6566, -63.6923) knots 0 0 0 0 1 1 1 1